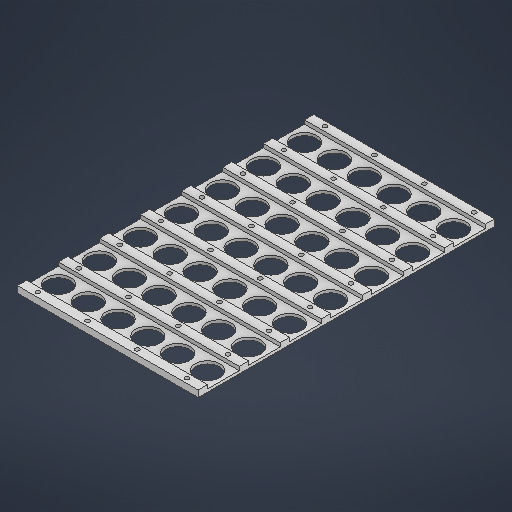
# Autodesk Inventor part: Chute
Saved by Autodesk Inventor 2025 (Build 290162010, 162A)
## iProperties
Created: 2025-12-04
Part Number: Chute
Material: Generic
Document SubType Name: Modeling
Designer: FizzyApple12
Density: 1 g/cm^3
Appearance: Default
Author: FizzyApple12
Autodesk Inventor part; units mm, degrees
ref_plane "YZ Plane" through (0, 0, 0) normal (1, 0, 0) x (0, 1, 0)
ref_plane "XZ Plane" through (0, 0, 0) normal (0, 1, 0) x (-1, 0, 0)
ref_plane "XY Plane" through (0, 0, 0) normal (0, 0, 1) x (1, 0, 0)
sketch "Sketch1" plane through (0, 0, 0) normal (0, 1, 0) x (-1, 0, 0)
  circle A0 centre (0, 0) radius 13
  line L0 (0, 0) -> (0, -264) construction
  line L1 (0, 0) -> (160, 0) construction
  circle A1 centre (0, -44) radius 13
  circle A2 centre (0, -88) radius 13
  circle A3 centre (0, -132) radius 13
  circle A4 centre (0, -176) radius 13
  circle A5 centre (0, -220) radius 13
  circle A6 centre (0, -264) radius 13
  circle A7 centre (32, 0) radius 13
  circle A8 centre (32, -44) radius 13
  circle A9 centre (32, -88) radius 13
  circle A10 centre (32, -132) radius 13
  circle A11 centre (32, -176) radius 13
  circle A12 centre (32, -220) radius 13
  circle A13 centre (32, -264) radius 13
  circle A14 centre (64, 0) radius 13
  circle A15 centre (64, -44) radius 13
  circle A16 centre (64, -88) radius 13
  circle A17 centre (64, -132) radius 13
  circle A18 centre (64, -176) radius 13
  circle A19 centre (64, -220) radius 13
  circle A20 centre (64, -264) radius 13
  circle A21 centre (96, 0) radius 13
  circle A22 centre (96, -44) radius 13
  circle A23 centre (96, -88) radius 13
  circle A24 centre (96, -132) radius 13
  circle A25 centre (96, -176) radius 13
  circle A26 centre (96, -220) radius 13
  circle A27 centre (96, -264) radius 13
  circle A28 centre (128, 0) radius 13
  circle A29 centre (128, -44) radius 13
  circle A30 centre (128, -88) radius 13
  circle A31 centre (128, -132) radius 13
  circle A32 centre (128, -176) radius 13
  circle A33 centre (128, -220) radius 13
  circle A34 centre (128, -264) radius 13
  circle A35 centre (160, 0) radius 13
  circle A36 centre (160, -44) radius 13
  circle A37 centre (160, -88) radius 13
  circle A38 centre (160, -132) radius 13
  circle A39 centre (160, -176) radius 13
  circle A40 centre (160, -220) radius 13
  circle A41 centre (160, -264) radius 13
  line L2 (-17, 27) -> (177, 27)
  line L3 (177, 27) -> (177, -291)
  line L4 (177, -291) -> (-17, -291)
  line L5 (-17, -291) -> (-17, 27)
  line L6 (-17, -17) -> (177, -17)
  line L7 (177, -17) -> (177, -27) construction
  line L8 (177, -27) -> (-17, -27)
  line L9 (-17, -27) -> (-17, -17) construction
  circle A42 centre (0.064, 22) radius 2.25 construction
  line L10 (177, 17) -> (-17, 17)
  line L11 (177, 17) -> (-17, -17) construction
  line L12 (-17, -281) -> (177, -281)
  line L13 (-17, -61) -> (177, -61)
  line L14 (177, -71) -> (-17, -71)
  line L15 (-17, -105) -> (177, -105)
  line L16 (177, -115) -> (-17, -115)
  line L17 (-17, -149) -> (177, -149)
  line L18 (177, -159) -> (-17, -159)
  line L19 (-17, -193) -> (177, -193)
  line L20 (177, -203) -> (-17, -203)
  line L21 (-17, -237) -> (177, -237)
  line L22 (177, -247) -> (-17, -247)
  line L23 (160, 0) -> (160, -44) construction
  line L24 (160, -22) -> (177, -22) construction
  point P0 (0.064, -22)
  point P1 (0.064, -66)
  point P2 (0.064, -110)
  point P3 (0.064, -154)
  point P4 (0.064, -198)
  point P5 (53.376, 22)
  point P6 (53.376, -22)
  point P7 (53.376, -66)
  point P8 (53.376, -110)
  point P9 (53.376, -154)
  point P10 (53.376, -198)
  point P11 (106.688, 22)
  point P12 (106.688, -22)
  point P13 (106.688, -66)
  point P14 (106.688, -110)
  point P15 (106.688, -154)
  point P16 (106.688, -198)
  point P17 (106.688, -22)
  point P18 (80, 0)
  point P19 (0.064, -242)
  point P20 (53.376, -242)
  point P21 (106.688, -242)
  point P22 (0.064, -22)
  point P23 (0.064, -286)
  point P24 (53.376, -286)
  point P25 (106.688, -286)
  point P26 (53.376, -22)
  point P27 (-17, -27)
  point P28 (-17, -71)
  point P29 (177, -71)
  point P30 (-17, -115)
  point P31 (177, -115)
  point P32 (-17, -159)
  point P33 (177, -159)
  point P34 (-17, -203)
  point P35 (177, -203)
  point P36 (-17, -247)
  point P37 (177, -247)
  point P38 (160, 22)
  point P39 (160, -66)
  point P40 (160, -110)
  point P41 (160, -154)
  point P42 (160, -198)
  point P43 (160, -242)
  point P44 (160, -286)
  dimension "d0" = 26
  dimension "d3" = 44
  dimension "d6" = 32
  dimension "d9" = 17
  dimension "d12" = 44
  dimension "d15" = 53.312
  dimension "d18" = 17
  dimension "d19" = 4.5
  dimension "d20" = 34
  dimension "d21" = 10
  dimension "d22" = 10
  dimension "d23" = 10
  dimension "d26" = 44
  dimension "d31" = 34
  constraints: 50 coincident, 50 end point, 43 centre point, 6 point on line, 5 horizontal, 5 perpendicular, 5 vertical, 4 midpoint, 4 parallel, 184 other
  measures "d0" diameter of A0
  measures "d3" distance of L0.start A1.centre
  measures "d6" distance of L0.start A7.centre
  measures "d9" distance between parallel lines of L5 L0
  measures "d12" distance of point (0.064, 22) point (0.064, -22)
  measures "d15" distance of point (0.064, 22) point (53.376, 22)
  measures "d18" distance from line of L3 L1.end
  measures "d19" diameter of A42
  measures "d20" distance between parallel lines of L6 L10
  measures "d21" distance between parallel lines of L8 L6
  measures "d22" distance between parallel lines of L10 L2
  measures "d23" distance between parallel lines of L4 L12
  measures "d26" distance of L6.start L13.start
  measures "d31" distance between parallel lines of L12 L22
extrude "Extrusion1" add sketch "Sketch1" along normal blind 3
extrude "Extrusion2" add sketch "Sketch1" along normal blind 7 contours L2 L3 L10 L5 | L6 L3 L8 L5 | L13 L3 L14 L5 | L15 L3 L16 L5 | L17 L3 L18 L5 | L19 L3 L20 L5 | L21 L3 L22 L5 | L12 L3 L4 L5
hole "Hole1" at (-0.064, 0, 22) at (-0.064, 0, -22) at (-0.064, 0, -66) at (-0.064, 0, -110) at (-0.064, 0, -154) at (-0.064, 0, -198) at (-53.376, 0, 22) at (-53.376, 0, -22) at (-53.376, 0, -66) at (-53.376, 0, -110) at (-53.376, 0, -154) at (-53.376, 0, -198) at (-106.688, 0, 22) at (-106.688, 0, -22) at (-106.688, 0, -66) at (-106.688, 0, -110) at (-106.688, 0, -154) at (-106.688, 0, -198) at (-0.064, 0, -242) at (-53.376, 0, -242) at (-106.688, 0, -242) at (-0.064, 0, -286) at (-53.376, 0, -286) at (-106.688, 0, -286) at (-160, 0, -22) at (-160, 0, 22) at (-160, 0, -66) at (-160, 0, -110) at (-160, 0, -154) at (-160, 0, -198) at (-160, 0, -242) at (-160, 0, -286) direction (0, 1, 0) diameter 4.5 end through all
equation "\"d12\" = d3"
equation "\"d15\" = 1.666 * d6"
equation "\"d18\" = d9"
equation "\"d22\" = d21"
equation "\"d23\" = d21"
equation "\"d26\" = d3"
equation "\"d31\" = d20"
body "Solid1"
